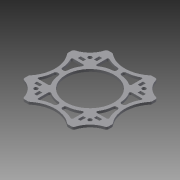
# Autodesk Inventor part: Plate1
Saved by Autodesk Inventor 2014 SP1 (Build 180222100, 222)
## iProperties
Created: 2014-07-27
Part Number: Plate1
Material: Generic
Document SubType Name: Modeling
Designer: Ryan
Density: 1 g/cm^3
Appearance: Default
Author: Ryan
Autodesk Inventor part; units mm, degrees
ref_plane "YZ Plane" through (0, 0, 0) normal (1, 0, 0) x (0, 1, 0)
ref_plane "XZ Plane" through (0, 0, 0) normal (0, 1, 0) x (-1, 0, 0)
ref_plane "XY Plane" through (0, 0, 0) normal (0, 0, 1) x (1, 0, 0)
sketch "Plate1" plane through (0, 0, 0) normal (0, 0, 1) x (1, 0, 0)
  line L0 (15.5481, 70) -> (18.2668, 70)
  line L1 (54.4519, 70) -> (51.7332, 70)
  arc A0 (19.5377, 69.5443) -> (50.4623, 69.5443) centre (35, 88.3333) ccw
  arc A1 (51.7332, 70) -> (50.4623, 69.5443) centre (51.7332, 68) ccw
  arc A2 (19.5377, 69.5443) -> (18.2668, 70) centre (18.2668, 68) ccw
  line L2 (70, 15.5481) -> (70, 18.2668)
  line L3 (70, 54.4519) -> (70, 51.7332)
  arc A3 (69.5443, 50.4623) -> (69.5443, 19.5377) centre (88.3333, 35) ccw
  arc A4 (70, 18.2668) -> (69.5443, 19.5377) centre (68, 18.2668) ccw
  arc A5 (69.5443, 50.4623) -> (70, 51.7332) centre (68, 51.7332) ccw
  line L4 (0, 54.4519) -> (0, 51.7332)
  line L5 (0, 15.5481) -> (0, 18.2668)
  arc A6 (0.4557, 19.5377) -> (0.4557, 50.4623) centre (-18.3333, 35) ccw
  arc A7 (0, 51.7332) -> (0.4557, 50.4623) centre (2, 51.7332) ccw
  arc A8 (0.4557, 19.5377) -> (0, 18.2668) centre (2, 18.2668) ccw
  line L6 (54.4519, 0) -> (51.7332, 0)
  line L7 (15.5481, 0) -> (18.2668, 0)
  arc A9 (50.4623, 0.4557) -> (19.5377, 0.4557) centre (35, -18.3333) ccw
  arc A10 (18.2668, 0) -> (19.5377, 0.4557) centre (18.2668, 2) ccw
  arc A11 (50.4623, 0.4557) -> (51.7332, 0) centre (51.7332, 2) ccw
  arc A12 (1.4232, 56.3669) -> (13.6331, 68.5768) centre (-3.8401, 73.8401) ccw
  arc A13 (1.4232, 56.3669) -> (0, 54.4519) centre (2, 54.4519) ccw
  arc A14 (15.5481, 70) -> (13.6331, 68.5768) centre (15.5481, 68) ccw
  arc A15 (68.5768, 13.6331) -> (56.3669, 1.4232) centre (73.8401, -3.8401) ccw
  arc A16 (68.5768, 13.6331) -> (70, 15.5481) centre (68, 15.5481) ccw
  arc A17 (54.4519, 0) -> (56.3669, 1.4232) centre (54.4519, 2) ccw
  arc A18 (56.3669, 68.5768) -> (68.5768, 56.3669) centre (73.8401, 73.8401) ccw
  arc A19 (56.3669, 68.5768) -> (54.4519, 70) centre (54.4519, 68) ccw
  arc A20 (70, 54.4519) -> (68.5768, 56.3669) centre (68, 54.4519) ccw
  arc A21 (13.6331, 1.4232) -> (1.4232, 13.6331) centre (-3.8401, -3.8401) ccw
  arc A22 (0, 15.5481) -> (1.4232, 13.6331) centre (2, 15.5481) ccw
  arc A23 (13.6331, 1.4232) -> (15.5481, 0) centre (15.5481, 2) ccw
  circle A24 centre (35, 35) radius 20
  line L8 (7.9, 52) -> (7.9, 54.4)
  line L9 (7.9, 54.4) -> (12.3, 54.4)
  line L10 (12.3, 54.4) -> (12.3, 52)
  line L11 (12.3, 52) -> (7.9, 52)
  line L12 (62.1, 54.4) -> (57.7, 54.4)
  line L13 (57.7, 54.4) -> (57.7, 51.9999)
  line L14 (57.7, 51.9999) -> (62.1, 52)
  line L15 (62.1, 52) -> (62.1, 54.4)
  line L16 (7.9, 18) -> (7.9, 15.6)
  line L17 (7.9, 15.6) -> (12.3, 15.6)
  line L18 (7.9, 18) -> (12.3, 18)
  line L19 (12.3, 18) -> (12.3, 15.6)
  line L20 (62.1, 18) -> (62.1, 15.6)
  line L21 (62.1, 15.6) -> (57.7, 15.6)
  line L22 (62.1, 18) -> (57.7, 18)
  line L23 (57.7, 18) -> (57.7, 15.6)
  line L24 (15.6, 62.1) -> (18, 62.1)
  line L25 (18, 62.1) -> (18, 57.7)
  line L26 (15.6, 62.1) -> (15.6, 57.7)
  line L27 (15.6, 57.7) -> (18, 57.7)
  line L28 (52, 62.1) -> (54.4, 62.1)
  line L29 (54.4, 62.1) -> (54.4, 57.7)
  line L30 (52, 62.1) -> (52, 57.7)
  line L31 (52, 57.7) -> (54.4, 57.7)
  line L32 (52, 7.9) -> (54.4, 7.9)
  line L33 (54.4, 7.9) -> (54.4, 12.3)
  line L34 (52, 7.9) -> (52, 12.3)
  line L35 (52, 12.3) -> (54.4, 12.3)
  line L36 (15.6, 7.9) -> (18, 7.9)
  line L37 (18, 7.9) -> (18, 12.3)
  line L38 (15.6, 7.9) -> (15.6, 12.3)
  line L39 (15.6, 12.3) -> (18, 12.3)
  line L40 (20.3865, 55.1716) -> (20.3865, 63.4714)
  arc A25 (21.8609, 64.3517) -> (31.5769, 61.6324) centre (32.759, 84.5725) ccw
  arc A26 (21.8609, 64.3517) -> (20.3865, 63.4714) centre (21.3865, 63.4714) ccw
  arc A27 (32.9998, 60.1341) -> (31.5769, 61.6324) centre (31.4998, 60.1343) ccw
  arc A28 (31.6146, 57.6251) -> (21.9333, 54.3343) centre (33.1944, 37.0907) ccw
  arc A29 (20.3865, 55.1716) -> (21.9333, 54.3343) centre (21.3865, 55.1716) ccw
  arc A30 (31.6146, 57.6251) -> (32.9996, 59.1204) centre (31.4996, 59.1206) ccw
  line L41 (32.9996, 59.1204) -> (32.9998, 60.1341)
  line L42 (49.6135, 55.1716) -> (49.6135, 63.4714)
  arc A31 (38.4231, 61.6324) -> (48.1391, 64.3517) centre (37.241, 84.5725) ccw
  arc A32 (49.6135, 63.4714) -> (48.1391, 64.3517) centre (48.6135, 63.4714) ccw
  arc A33 (38.4231, 61.6324) -> (37.0002, 60.1341) centre (38.5002, 60.1343) ccw
  arc A34 (48.0667, 54.3343) -> (38.3854, 57.6251) centre (36.8056, 37.0907) ccw
  arc A35 (48.0667, 54.3343) -> (49.6135, 55.1716) centre (48.6135, 55.1716) ccw
  arc A36 (37.0004, 59.1204) -> (38.3854, 57.6251) centre (38.5004, 59.1206) ccw
  line L43 (37.0004, 59.1204) -> (37.0002, 60.1341)
  line L44 (20.3865, 14.8284) -> (20.3865, 6.5286)
  arc A37 (31.5769, 8.3676) -> (21.8609, 5.6483) centre (32.759, -14.5725) ccw
  arc A38 (20.3865, 6.5286) -> (21.8609, 5.6483) centre (21.3865, 6.5286) ccw
  arc A39 (31.5769, 8.3676) -> (32.9998, 9.8659) centre (31.4998, 9.8657) ccw
  arc A40 (21.9333, 15.6657) -> (31.6146, 12.3749) centre (33.1944, 32.9093) ccw
  arc A41 (21.9333, 15.6657) -> (20.3865, 14.8284) centre (21.3865, 14.8284) ccw
  arc A42 (32.9996, 10.8796) -> (31.6146, 12.3749) centre (31.4996, 10.8794) ccw
  line L45 (32.9996, 10.8796) -> (32.9998, 9.8659)
  line L46 (49.6135, 14.8284) -> (49.6135, 6.5286)
  arc A43 (48.1391, 5.6483) -> (38.4231, 8.3676) centre (37.241, -14.5725) ccw
  arc A44 (48.1391, 5.6483) -> (49.6135, 6.5286) centre (48.6135, 6.5286) ccw
  arc A45 (37.0002, 9.8659) -> (38.4231, 8.3676) centre (38.5002, 9.8657) ccw
  arc A46 (38.3854, 12.3749) -> (48.0667, 15.6657) centre (36.8056, 32.9093) ccw
  arc A47 (49.6135, 14.8284) -> (48.0667, 15.6657) centre (48.6135, 14.8284) ccw
  arc A48 (38.3854, 12.3749) -> (37.0004, 10.8796) centre (38.5004, 10.8794) ccw
  line L47 (37.0004, 10.8796) -> (37.0002, 9.8659)
  line L48 (55.1716, 20.3865) -> (63.4714, 20.3865)
  arc A49 (61.6324, 31.5769) -> (64.3517, 21.8609) centre (84.5725, 32.759) ccw
  arc A50 (63.4714, 20.3865) -> (64.3517, 21.8609) centre (63.4714, 21.3865) ccw
  arc A51 (61.6324, 31.5769) -> (60.1341, 32.9998) centre (60.1343, 31.4998) ccw
  arc A52 (54.3343, 21.9333) -> (57.6251, 31.6146) centre (37.0907, 33.1944) ccw
  arc A53 (54.3343, 21.9333) -> (55.1716, 20.3865) centre (55.1716, 21.3865) ccw
  arc A54 (59.1204, 32.9996) -> (57.6251, 31.6146) centre (59.1206, 31.4996) ccw
  line L49 (59.1204, 32.9996) -> (60.1341, 32.9998)
  line L50 (55.1716, 49.6135) -> (63.4714, 49.6135)
  arc A55 (64.3517, 48.1391) -> (61.6324, 38.4231) centre (84.5725, 37.241) ccw
  arc A56 (64.3517, 48.1391) -> (63.4714, 49.6135) centre (63.4714, 48.6135) ccw
  arc A57 (60.1341, 37.0002) -> (61.6324, 38.4231) centre (60.1343, 38.5002) ccw
  arc A58 (57.6251, 38.3854) -> (54.3343, 48.0667) centre (37.0907, 36.8056) ccw
  arc A59 (55.1716, 49.6135) -> (54.3343, 48.0667) centre (55.1716, 48.6135) ccw
  arc A60 (57.6251, 38.3854) -> (59.1204, 37.0004) centre (59.1206, 38.5004) ccw
  line L51 (59.1204, 37.0004) -> (60.1341, 37.0002)
  line L52 (14.8284, 49.6135) -> (6.5286, 49.6135)
  arc A61 (8.3676, 38.4231) -> (5.6483, 48.1391) centre (-14.5725, 37.241) ccw
  arc A62 (6.5286, 49.6135) -> (5.6483, 48.1391) centre (6.5286, 48.6135) ccw
  arc A63 (8.3676, 38.4231) -> (9.8659, 37.0002) centre (9.8657, 38.5002) ccw
  arc A64 (15.6657, 48.0667) -> (12.3749, 38.3854) centre (32.9093, 36.8056) ccw
  arc A65 (15.6657, 48.0667) -> (14.8284, 49.6135) centre (14.8284, 48.6135) ccw
  arc A66 (10.8796, 37.0004) -> (12.3749, 38.3854) centre (10.8794, 38.5004) ccw
  line L53 (10.8796, 37.0004) -> (9.8659, 37.0002)
  line L54 (14.8284, 20.3865) -> (6.5286, 20.3865)
  arc A67 (5.6483, 21.8609) -> (8.3676, 31.5769) centre (-14.5725, 32.759) ccw
  arc A68 (5.6483, 21.8609) -> (6.5286, 20.3865) centre (6.5286, 21.3865) ccw
  arc A69 (9.8659, 32.9998) -> (8.3676, 31.5769) centre (9.8657, 31.4998) ccw
  arc A70 (12.3749, 31.6146) -> (15.6657, 21.9333) centre (32.9093, 33.1944) ccw
  arc A71 (14.8284, 20.3865) -> (15.6657, 21.9333) centre (14.8284, 21.3865) ccw
  arc A72 (12.3749, 31.6146) -> (10.8796, 32.9996) centre (10.8794, 31.4996) ccw
  line L55 (10.8796, 32.9996) -> (9.8659, 32.9998)
  circle A73 centre (12.5, 12.5) radius 1.6
  circle A74 centre (12.5, 57.5) radius 1.6
  circle A75 centre (57.5, 57.5) radius 1.6
  circle A76 centre (57.5, 12.5) radius 1.6
  point P0 (35, 35)
sketch "Sketch1" plane through (0, 0, 0) normal (0, 1, 0) x (-1, 0, 0)
  circle A0 centre (35, 35) radius 20
  arc A1 (1.4232, 56.3669) -> (13.6331, 68.5768) centre (-3.8401, 73.8401) ccw
  arc A2 (19.5377, 69.5443) -> (50.4623, 69.5443) centre (35, 88.3333) ccw
  arc A3 (56.3669, 68.5768) -> (68.5768, 56.3669) centre (73.8401, 73.8401) ccw
  arc A4 (69.5443, 50.4623) -> (69.5443, 19.5377) centre (88.3333, 35) ccw
  arc A5 (68.5768, 13.6331) -> (56.3669, 1.4232) centre (73.8401, -3.8401) ccw
  arc A6 (50.4623, 0.4557) -> (19.5377, 0.4557) centre (35, -18.3333) ccw
  arc A7 (13.6331, 1.4232) -> (1.4232, 13.6331) centre (-3.8401, -3.8401) ccw
  arc A8 (0.4557, 19.5377) -> (0.4557, 50.4623) centre (-18.3333, 35) ccw
  arc A9 (19.5377, 69.5443) -> (18.2668, 70) centre (18.2668, 68) ccw
  arc A10 (15.5481, 70) -> (13.6331, 68.5768) centre (15.5481, 68) ccw
  arc A11 (1.4232, 56.3669) -> (0, 54.4519) centre (2, 54.4519) ccw
  arc A12 (0, 51.7332) -> (0.4557, 50.4623) centre (2, 51.7332) ccw
  arc A13 (0.4557, 19.5377) -> (0, 18.2668) centre (2, 18.2668) ccw
  arc A14 (0, 15.5481) -> (1.4232, 13.6331) centre (2, 15.5481) ccw
  arc A15 (18.2668, 0) -> (19.5377, 0.4557) centre (18.2668, 2) ccw
  arc A16 (13.6331, 1.4232) -> (15.5481, 0) centre (15.5481, 2) ccw
  arc A17 (54.4519, 0) -> (56.3669, 1.4232) centre (54.4519, 2) ccw
  arc A18 (50.4623, 0.4557) -> (51.7332, 0) centre (51.7332, 2) ccw
  arc A19 (70, 18.2668) -> (69.5443, 19.5377) centre (68, 18.2668) ccw
  arc A20 (68.5768, 13.6331) -> (70, 15.5481) centre (68, 15.5481) ccw
  arc A21 (70, 54.4519) -> (68.5768, 56.3669) centre (68, 54.4519) ccw
  arc A22 (69.5443, 50.4623) -> (70, 51.7332) centre (68, 51.7332) ccw
  arc A23 (51.7332, 70) -> (50.4623, 69.5443) centre (51.7332, 68) ccw
  arc A24 (56.3669, 68.5768) -> (54.4519, 70) centre (54.4519, 68) ccw
  line L0 (0, 15.5481) -> (0, 18.2668)
  line L1 (15.5481, 0) -> (18.2668, 0)
  line L2 (51.7332, 0) -> (54.4519, 0)
  line L3 (70, 15.5481) -> (70, 18.2668)
  line L4 (70, 51.7332) -> (70, 54.4519)
  line L5 (54.4519, 70) -> (51.7332, 70)
  line L6 (18.2668, 70) -> (15.5481, 70)
  line L7 (0, 54.2922) -> (0, 51.7332)
  circle A25 centre (12.5, 57.5) radius 1.6
  circle A26 centre (57.5, 57.5) radius 1.6
  circle A27 centre (57.5, 12.5) radius 1.6
  circle A28 centre (12.5, 12.5) radius 1.6
  line L8 (7.9, 54.4) -> (12.3, 54.4)
  line L9 (12.3, 54.4) -> (12.3, 52)
  line L10 (12.3, 52) -> (7.9, 52)
  line L11 (7.9, 52) -> (7.9, 54.4)
  line L12 (15.6, 62.1) -> (18, 62.1)
  line L13 (18, 62.1) -> (18, 57.7)
  line L14 (18, 57.7) -> (15.6, 57.7)
  line L15 (15.6, 57.7) -> (15.6, 62.1)
  line L16 (52, 62.1) -> (54.4, 62.1)
  line L17 (54.4, 62.1) -> (54.4, 57.7)
  line L18 (54.4, 57.7) -> (52, 57.7)
  line L19 (52, 57.7) -> (52, 62.1)
  line L20 (57.7, 54.4) -> (62.1, 54.4)
  line L21 (62.1, 54.4) -> (62.1, 52)
  line L22 (62.1, 52) -> (57.7, 52)
  line L23 (57.7, 52) -> (57.7, 54.4)
  line L24 (57.7, 18) -> (62.1, 18)
  line L25 (62.1, 18) -> (62.1, 15.6)
  line L26 (62.1, 15.6) -> (57.7, 15.6)
  line L27 (57.7, 15.6) -> (57.7, 18)
  line L28 (52, 12.3) -> (54.4, 12.3)
  line L29 (54.4, 12.3) -> (54.4, 7.9)
  line L30 (54.4, 7.9) -> (52, 7.9)
  line L31 (52, 7.9) -> (52, 12.3)
  line L32 (15.6, 12.3) -> (18, 12.3)
  line L33 (18, 12.3) -> (18, 7.9)
  line L34 (18, 7.9) -> (15.6, 7.9)
  line L35 (15.6, 7.9) -> (15.6, 12.3)
  line L36 (7.9, 18) -> (12.3, 18)
  line L37 (12.3, 18) -> (12.3, 15.6)
  line L38 (12.3, 15.6) -> (7.9, 15.6)
  line L39 (7.9, 15.6) -> (7.9, 18)
  arc A29 (32.9998, 60.1341) -> (31.5769, 61.6324) centre (31.4998, 60.1343) ccw
  arc A30 (38.4231, 61.6324) -> (37.0002, 60.1341) centre (38.5002, 60.1343) ccw
  arc A31 (37.0004, 59.1204) -> (38.3854, 57.6251) centre (38.5004, 59.1206) ccw
  arc A32 (49.6135, 63.4714) -> (48.1391, 64.3517) centre (48.6135, 63.4714) ccw
  arc A33 (48.0667, 54.3343) -> (49.6135, 55.1716) centre (48.6135, 55.1716) ccw
  arc A34 (20.3865, 55.1716) -> (21.9333, 54.3343) centre (21.3865, 55.1716) ccw
  arc A35 (21.8609, 64.3517) -> (20.3865, 63.4714) centre (21.3865, 63.4714) ccw
  arc A36 (55.1716, 49.6135) -> (54.3343, 48.0667) centre (55.1716, 48.6135) ccw
  arc A37 (64.3517, 48.1391) -> (63.4714, 49.6135) centre (63.4714, 48.6135) ccw
  arc A38 (60.1341, 37.0002) -> (61.6324, 38.4231) centre (60.1343, 38.5002) ccw
  arc A39 (57.6251, 38.3854) -> (59.1204, 37.0004) centre (59.1206, 38.5004) ccw
  arc A40 (59.1204, 32.9996) -> (57.6251, 31.6146) centre (59.1206, 31.4996) ccw
  arc A41 (61.6324, 31.5769) -> (60.1341, 32.9998) centre (60.1343, 31.4998) ccw
  arc A42 (63.4714, 20.3865) -> (64.3517, 21.8609) centre (63.4714, 21.3865) ccw
  arc A43 (54.3343, 21.9333) -> (55.1716, 20.3865) centre (55.1716, 21.3865) ccw
  arc A44 (49.6135, 14.8284) -> (48.0667, 15.6657) centre (48.6135, 14.8284) ccw
  arc A45 (48.1391, 5.6483) -> (49.6135, 6.5286) centre (48.6135, 6.5286) ccw
  arc A46 (37.0002, 9.8659) -> (38.4231, 8.3676) centre (38.5002, 9.8657) ccw
  arc A47 (38.3854, 12.3749) -> (37.0004, 10.8796) centre (38.5004, 10.8794) ccw
  arc A48 (31.5769, 8.3676) -> (32.9998, 9.8659) centre (31.4998, 9.8657) ccw
  arc A49 (32.9996, 10.8796) -> (31.6146, 12.3749) centre (31.4996, 10.8794) ccw
  arc A50 (21.9333, 15.6657) -> (20.3865, 14.8284) centre (21.3865, 14.8284) ccw
  arc A51 (20.3865, 6.5286) -> (21.8609, 5.6483) centre (21.3865, 6.5286) ccw
  arc A52 (5.6483, 21.8609) -> (6.5286, 20.3865) centre (6.5286, 21.3865) ccw
  arc A53 (14.8284, 20.3865) -> (15.6657, 21.9333) centre (14.8284, 21.3865) ccw
  arc A54 (12.3749, 31.6146) -> (10.8796, 32.9996) centre (10.8794, 31.4996) ccw
  arc A55 (9.8659, 32.9998) -> (8.3676, 31.5769) centre (9.8657, 31.4998) ccw
  arc A56 (6.5286, 49.6135) -> (5.6483, 48.1391) centre (6.5286, 48.6135) ccw
  arc A57 (15.6657, 48.0667) -> (14.8284, 49.6135) centre (14.8284, 48.6135) ccw
  arc A58 (10.8796, 37.0004) -> (12.3749, 38.3854) centre (10.8794, 38.5004) ccw
  arc A59 (8.3676, 38.4231) -> (9.8659, 37.0002) centre (9.8657, 38.5002) ccw
  arc A60 (31.6146, 57.6251) -> (32.9996, 59.1204) centre (31.4996, 59.1206) ccw
  arc A61 (5.6483, 21.8609) -> (8.3676, 31.5769) centre (-14.5725, 32.759) ccw
  arc A62 (12.3749, 31.6146) -> (15.6657, 21.9333) centre (32.9093, 33.1944) ccw
  arc A63 (15.6657, 48.0667) -> (12.3749, 38.3854) centre (32.9093, 36.8056) ccw
  arc A64 (8.3676, 38.4231) -> (5.6483, 48.1391) centre (-14.5725, 37.241) ccw
  line L40 (6.5286, 20.3865) -> (14.8284, 20.3865)
  line L41 (10.8796, 32.9996) -> (9.8659, 32.9998)
  line L42 (9.8659, 37.0002) -> (10.8796, 37.0004)
  line L43 (6.5286, 49.6135) -> (14.8284, 49.6135)
  arc A65 (21.9333, 15.6657) -> (31.6146, 12.3749) centre (33.1944, 32.9093) ccw
  arc A66 (38.3854, 12.3749) -> (48.0667, 15.6657) centre (36.8056, 32.9093) ccw
  arc A67 (48.0667, 54.3343) -> (38.3854, 57.6251) centre (36.8056, 37.0907) ccw
  arc A68 (31.6146, 57.6251) -> (21.9333, 54.3343) centre (33.1944, 37.0907) ccw
  arc A69 (57.6251, 38.3854) -> (54.3343, 48.0667) centre (37.0907, 36.8056) ccw
  arc A70 (54.3343, 21.9333) -> (57.6251, 31.6146) centre (37.0907, 33.1944) ccw
  arc A71 (31.5769, 8.3676) -> (21.8609, 5.6483) centre (32.759, -14.5725) ccw
  arc A72 (48.1391, 5.6483) -> (38.4231, 8.3676) centre (37.241, -14.5725) ccw
  arc A73 (61.6324, 31.5769) -> (64.3517, 21.8609) centre (84.5725, 32.759) ccw
  arc A74 (64.3517, 48.1391) -> (61.6324, 38.4231) centre (84.5725, 37.241) ccw
  arc A75 (21.8609, 64.3517) -> (31.5769, 61.6324) centre (32.759, 84.5725) ccw
  arc A76 (38.4231, 61.6324) -> (48.1391, 64.3517) centre (37.241, 84.5725) ccw
  line L44 (20.3865, 14.8284) -> (20.3865, 6.5286)
  line L45 (32.9996, 10.8796) -> (32.9998, 9.8659)
  line L46 (37.0004, 10.8796) -> (37.0002, 9.8659)
  line L47 (49.6135, 14.8284) -> (49.6135, 6.5286)
  line L48 (55.1716, 20.3865) -> (63.4714, 20.3865)
  line L49 (59.1204, 32.9996) -> (60.1341, 32.9998)
  line L50 (59.1204, 37.0004) -> (60.1341, 37.0002)
  line L51 (55.1716, 49.6135) -> (63.4714, 49.6135)
  line L52 (49.6135, 63.4714) -> (49.6135, 55.1716)
  line L53 (37.0004, 59.1204) -> (37.0002, 60.1341)
  line L54 (32.9998, 60.1341) -> (32.9996, 59.1204)
  line L55 (20.3865, 63.4714) -> (20.3865, 55.1716)
  line L56 (0, 54.2922) -> (0, 54.4519)
  line L57 (15.5481, 70) -> (18.2668, 70)
  line L58 (54.4519, 70) -> (51.7332, 70)
  arc A77 (19.5377, 69.5443) -> (50.4623, 69.5443) centre (35, 88.3333) ccw
  arc A78 (51.7332, 70) -> (50.4623, 69.5443) centre (51.7332, 68) ccw
  arc A79 (19.5377, 69.5443) -> (18.2668, 70) centre (18.2668, 68) ccw
  line L59 (70, 15.5481) -> (70, 18.2668)
  line L60 (70, 54.4519) -> (70, 51.7332)
  arc A80 (69.5443, 50.4623) -> (69.5443, 19.5377) centre (88.3333, 35) ccw
  arc A81 (70, 18.2668) -> (69.5443, 19.5377) centre (68, 18.2668) ccw
  arc A82 (69.5443, 50.4623) -> (70, 51.7332) centre (68, 51.7332) ccw
  line L61 (0, 54.4519) -> (0, 51.7332)
  line L62 (0, 15.5481) -> (0, 18.2668)
  arc A83 (0.4557, 19.5377) -> (0.4557, 50.4623) centre (-18.3333, 35) ccw
  arc A84 (0, 51.7332) -> (0.4557, 50.4623) centre (2, 51.7332) ccw
  arc A85 (0.4557, 19.5377) -> (0, 18.2668) centre (2, 18.2668) ccw
  line L63 (54.4519, 0) -> (51.7332, 0)
  line L64 (15.5481, 0) -> (18.2668, 0)
  arc A86 (50.4623, 0.4557) -> (19.5377, 0.4557) centre (35, -18.3333) ccw
  arc A87 (18.2668, 0) -> (19.5377, 0.4557) centre (18.2668, 2) ccw
  arc A88 (50.4623, 0.4557) -> (51.7332, 0) centre (51.7332, 2) ccw
  arc A89 (1.4232, 56.3669) -> (13.6331, 68.5768) centre (-3.8401, 73.8401) ccw
  arc A90 (1.4232, 56.3669) -> (0, 54.4519) centre (2, 54.4519) ccw
  arc A91 (15.5481, 70) -> (13.6331, 68.5768) centre (15.5481, 68) ccw
  arc A92 (68.5768, 13.6331) -> (56.3669, 1.4232) centre (73.8401, -3.8401) ccw
  arc A93 (68.5768, 13.6331) -> (70, 15.5481) centre (68, 15.5481) ccw
  arc A94 (54.4519, 0) -> (56.3669, 1.4232) centre (54.4519, 2) ccw
  arc A95 (56.3669, 68.5768) -> (68.5768, 56.3669) centre (73.8401, 73.8401) ccw
  arc A96 (56.3669, 68.5768) -> (54.4519, 70) centre (54.4519, 68) ccw
  arc A97 (70, 54.4519) -> (68.5768, 56.3669) centre (68, 54.4519) ccw
  arc A98 (13.6331, 1.4232) -> (1.4232, 13.6331) centre (-3.8401, -3.8401) ccw
  arc A99 (0, 15.5481) -> (1.4232, 13.6331) centre (2, 15.5481) ccw
  arc A100 (13.6331, 1.4232) -> (15.5481, 0) centre (15.5481, 2) ccw
  circle A101 centre (35, 35) radius 20
  line L65 (7.9, 52) -> (7.9, 54.4)
  line L66 (7.9, 54.4) -> (12.3, 54.4)
  line L67 (12.3, 54.4) -> (12.3, 52)
  line L68 (12.3, 52) -> (7.9, 52)
  line L69 (62.1, 54.4) -> (57.7, 54.4)
  line L70 (57.7, 54.4) -> (57.7, 51.9999)
  line L71 (57.7, 51.9999) -> (62.1, 52)
  line L72 (62.1, 52) -> (62.1, 54.4)
  line L73 (7.9, 18) -> (7.9, 15.6)
  line L74 (7.9, 15.6) -> (12.3, 15.6)
  line L75 (7.9, 18) -> (12.3, 18)
  line L76 (12.3, 18) -> (12.3, 15.6)
  line L77 (62.1, 18) -> (62.1, 15.6)
  line L78 (62.1, 15.6) -> (57.7, 15.6)
  line L79 (62.1, 18) -> (57.7, 18)
  line L80 (57.7, 18) -> (57.7, 15.6)
  line L81 (15.6, 62.1) -> (18, 62.1)
  line L82 (18, 62.1) -> (18, 57.7)
  line L83 (15.6, 62.1) -> (15.6, 57.7)
  line L84 (15.6, 57.7) -> (18, 57.7)
  line L85 (52, 62.1) -> (54.4, 62.1)
  line L86 (54.4, 62.1) -> (54.4, 57.7)
  line L87 (52, 62.1) -> (52, 57.7)
  line L88 (52, 57.7) -> (54.4, 57.7)
  line L89 (52, 7.9) -> (54.4, 7.9)
  line L90 (54.4, 7.9) -> (54.4, 12.3)
  line L91 (52, 7.9) -> (52, 12.3)
  line L92 (52, 12.3) -> (54.4, 12.3)
  line L93 (15.6, 7.9) -> (18, 7.9)
  line L94 (18, 7.9) -> (18, 12.3)
  line L95 (15.6, 7.9) -> (15.6, 12.3)
  line L96 (15.6, 12.3) -> (18, 12.3)
  line L97 (20.3865, 55.1716) -> (20.3865, 63.4714)
  arc A102 (21.8609, 64.3517) -> (31.5769, 61.6324) centre (32.759, 84.5725) ccw
  arc A103 (21.8609, 64.3517) -> (20.3865, 63.4714) centre (21.3865, 63.4714) ccw
  arc A104 (32.9998, 60.1341) -> (31.5769, 61.6324) centre (31.4998, 60.1343) ccw
  arc A105 (31.6146, 57.6251) -> (21.9333, 54.3343) centre (33.1944, 37.0907) ccw
  arc A106 (20.3865, 55.1716) -> (21.9333, 54.3343) centre (21.3865, 55.1716) ccw
  arc A107 (31.6146, 57.6251) -> (32.9996, 59.1204) centre (31.4996, 59.1206) ccw
  line L98 (32.9996, 59.1204) -> (32.9998, 60.1341)
  line L99 (49.6135, 55.1716) -> (49.6135, 63.4714)
  arc A108 (38.4231, 61.6324) -> (48.1391, 64.3517) centre (37.241, 84.5725) ccw
  arc A109 (49.6135, 63.4714) -> (48.1391, 64.3517) centre (48.6135, 63.4714) ccw
  arc A110 (38.4231, 61.6324) -> (37.0002, 60.1341) centre (38.5002, 60.1343) ccw
  arc A111 (48.0667, 54.3343) -> (38.3854, 57.6251) centre (36.8056, 37.0907) ccw
  arc A112 (48.0667, 54.3343) -> (49.6135, 55.1716) centre (48.6135, 55.1716) ccw
  arc A113 (37.0004, 59.1204) -> (38.3854, 57.6251) centre (38.5004, 59.1206) ccw
  line L100 (37.0004, 59.1204) -> (37.0002, 60.1341)
  line L101 (20.3865, 14.8284) -> (20.3865, 6.5286)
  arc A114 (31.5769, 8.3676) -> (21.8609, 5.6483) centre (32.759, -14.5725) ccw
  arc A115 (20.3865, 6.5286) -> (21.8609, 5.6483) centre (21.3865, 6.5286) ccw
  arc A116 (31.5769, 8.3676) -> (32.9998, 9.8659) centre (31.4998, 9.8657) ccw
  arc A117 (21.9333, 15.6657) -> (31.6146, 12.3749) centre (33.1944, 32.9093) ccw
  arc A118 (21.9333, 15.6657) -> (20.3865, 14.8284) centre (21.3865, 14.8284) ccw
  arc A119 (32.9996, 10.8796) -> (31.6146, 12.3749) centre (31.4996, 10.8794) ccw
  line L102 (32.9996, 10.8796) -> (32.9998, 9.8659)
  line L103 (49.6135, 14.8284) -> (49.6135, 6.5286)
  arc A120 (48.1391, 5.6483) -> (38.4231, 8.3676) centre (37.241, -14.5725) ccw
  arc A121 (48.1391, 5.6483) -> (49.6135, 6.5286) centre (48.6135, 6.5286) ccw
  arc A122 (37.0002, 9.8659) -> (38.4231, 8.3676) centre (38.5002, 9.8657) ccw
  arc A123 (38.3854, 12.3749) -> (48.0667, 15.6657) centre (36.8056, 32.9093) ccw
  arc A124 (49.6135, 14.8284) -> (48.0667, 15.6657) centre (48.6135, 14.8284) ccw
  arc A125 (38.3854, 12.3749) -> (37.0004, 10.8796) centre (38.5004, 10.8794) ccw
  line L104 (37.0004, 10.8796) -> (37.0002, 9.8659)
  line L105 (55.1716, 20.3865) -> (63.4714, 20.3865)
  arc A126 (61.6324, 31.5769) -> (64.3517, 21.8609) centre (84.5725, 32.759) ccw
  arc A127 (63.4714, 20.3865) -> (64.3517, 21.8609) centre (63.4714, 21.3865) ccw
  arc A128 (61.6324, 31.5769) -> (60.1341, 32.9998) centre (60.1343, 31.4998) ccw
  arc A129 (54.3343, 21.9333) -> (57.6251, 31.6146) centre (37.0907, 33.1944) ccw
  arc A130 (54.3343, 21.9333) -> (55.1716, 20.3865) centre (55.1716, 21.3865) ccw
  arc A131 (59.1204, 32.9996) -> (57.6251, 31.6146) centre (59.1206, 31.4996) ccw
  line L106 (59.1204, 32.9996) -> (60.1341, 32.9998)
  line L107 (55.1716, 49.6135) -> (63.4714, 49.6135)
  arc A132 (64.3517, 48.1391) -> (61.6324, 38.4231) centre (84.5725, 37.241) ccw
  arc A133 (64.3517, 48.1391) -> (63.4714, 49.6135) centre (63.4714, 48.6135) ccw
  arc A134 (60.1341, 37.0002) -> (61.6324, 38.4231) centre (60.1343, 38.5002) ccw
  arc A135 (57.6251, 38.3854) -> (54.3343, 48.0667) centre (37.0907, 36.8056) ccw
  arc A136 (55.1716, 49.6135) -> (54.3343, 48.0667) centre (55.1716, 48.6135) ccw
  arc A137 (57.6251, 38.3854) -> (59.1204, 37.0004) centre (59.1206, 38.5004) ccw
  line L108 (59.1204, 37.0004) -> (60.1341, 37.0002)
  line L109 (14.8284, 49.6135) -> (6.5286, 49.6135)
  arc A138 (8.3676, 38.4231) -> (5.6483, 48.1391) centre (-14.5725, 37.241) ccw
  arc A139 (6.5286, 49.6135) -> (5.6483, 48.1391) centre (6.5286, 48.6135) ccw
  arc A140 (8.3676, 38.4231) -> (9.8659, 37.0002) centre (9.8657, 38.5002) ccw
  arc A141 (15.6657, 48.0667) -> (12.3749, 38.3854) centre (32.9093, 36.8056) ccw
  arc A142 (15.6657, 48.0667) -> (14.8284, 49.6135) centre (14.8284, 48.6135) ccw
  arc A143 (10.8796, 37.0004) -> (12.3749, 38.3854) centre (10.8794, 38.5004) ccw
  line L110 (10.8796, 37.0004) -> (9.8659, 37.0002)
  line L111 (14.8284, 20.3865) -> (6.5286, 20.3865)
  arc A144 (5.6483, 21.8609) -> (8.3676, 31.5769) centre (-14.5725, 32.759) ccw
  arc A145 (5.6483, 21.8609) -> (6.5286, 20.3865) centre (6.5286, 21.3865) ccw
  arc A146 (9.8659, 32.9998) -> (8.3676, 31.5769) centre (9.8657, 31.4998) ccw
  arc A147 (12.3749, 31.6146) -> (15.6657, 21.9333) centre (32.9093, 33.1944) ccw
  arc A148 (14.8284, 20.3865) -> (15.6657, 21.9333) centre (14.8284, 21.3865) ccw
  arc A149 (12.3749, 31.6146) -> (10.8796, 32.9996) centre (10.8794, 31.4996) ccw
  line L112 (10.8796, 32.9996) -> (9.8659, 32.9998)
  circle A150 centre (12.5, 12.5) radius 1.6
  circle A151 centre (12.5, 57.5) radius 1.6
  circle A152 centre (57.5, 57.5) radius 1.6
  circle A153 centre (57.5, 12.5) radius 1.6
  point P0 (0, 0)
  constraints: 144 point on circle, 114 end point, 77 centre point, 48 tangent, 29 horizontal, 22 vertical, 17 parallel, 11 perpendicular, 1 collinear, 220 other
extrude "Extrusion1" add sketch "Sketch1" along normal blind 2
body "Solid1"
